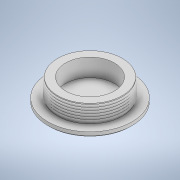
# Autodesk Inventor part: Abdeckung_Sensorkopfh
Saved by Autodesk Inventor 2022 (Build 260153000, 153)
## iProperties
Created: 2023-07-31
Part Number: Abdeckung_Sensorkopfh
Material: Generisch
Document SubType Name: Modeling
Designer: aewalder
Density: 1 g/cm^3
Appearance: Vorgabe
Author: aewalder
Autodesk Inventor part; units mm, degrees
ref_plane "YZ Plane" through (0, 0, 0) normal (1, 0, 0) x (0, 1, 0)
ref_plane "XZ Plane" through (0, 0, 0) normal (0, 1, 0) x (-1, 0, 0)
ref_plane "XY Plane" through (0, 0, 0) normal (0, 0, 1) x (1, 0, 0)
sketch "Sketch1" plane through (0, 0, 0) normal (0, 0, 1) x (1, 0, 0)
  line L0 (16, 0) -> (16, 1.8)
  line L1 (16, 1.8) -> (12.3, 1.8)
  line L2 (12.3, 1.8) -> (12.3, 2.4)
  arc A0 (12.3, 2.4) -> (12.3, 3.2) centre (12.3, 2.8) ccw
  line L3 (12.3, 3.2) -> (12.3, 3.4)
  arc A1 (12.3, 3.4) -> (12.3, 4.2) centre (12.3, 3.8) ccw
  line L4 (12.3, 4.2) -> (12.3, 4.4)
  arc A2 (12.3, 4.4) -> (12.3, 5.2) centre (12.3, 4.8) ccw
  line L5 (12.3, 5.2) -> (12.3, 8.6)
  line L6 (12.3, 8.6) -> (9.3, 8.6)
  line L7 (9.3, 8.6) -> (9.3, 1.8)
  line L8 (9.3, 1.8) -> (0, 1.8)
  line L9 (0, 1.8) -> (0, 0)
  line L10 (0, 0) -> (16, 0)
  line L11 (12.5, 4.8) -> (12.5, 2.8) construction
  line L12 (12.3, 4.8) -> (12.5, 4.8) construction
  line L13 (12.3, 2.8) -> (12.5, 2.8) construction
  line L14 (12.7, 4.8) -> (12.7, 2.8) construction
  line L15 (12.3, 5.8) -> (12.5, 5.8) construction
  arc A3 (12.3, 5.4) -> (12.3, 6.2) centre (12.3, 5.8) ccw
  line L16 (12.3, 6.8) -> (12.5, 6.8) construction
  arc A4 (12.3, 6.4) -> (12.3, 7.2) centre (12.3, 6.8) ccw
  line L17 (12.3, 7.8) -> (12.5, 7.8) construction
  arc A5 (12.3, 7.4) -> (12.3, 8.2) centre (12.3, 7.8) ccw
  point P0 (12.7, 5.8)
  point P1 (12.7, 6.8)
  point P2 (12.7, 7.8)
  point P3 (12.3, 8.2)
  point P4 (12.3, 7.4)
  point P5 (12.3, 6.2)
  point P6 (12.3, 5.4)
  point P7 (12.3, 7.2)
  point P8 (12.3, 6.4)
  dimension "d0" = 25
  dimension "d1" = 0.2
  dimension "d2" = 1
  dimension "d3" = 1
  dimension "d5" = 1
  dimension "d6" = 0.2
  dimension "d8" = 1.8
  dimension "d10" = 32
  dimension "d17" = 1
  dimension "d22" = 0.8
  dimension "d23" = 3
  constraints: 36 end point, 14 point on circle, 11 point on line, 6 centre point, 5 perpendicular, 3 horizontal, 3 vertical, 2 equal radius, 21 other
  measures "d0" diameter of L11 L9
  measures "d1" distance between parallel lines of L14 L11
  measures "d2" distance of L13.start A1.centre
  measures "d3" distance of L12.start A1.centre
  measures "d5" distance from line of L1 L13.start
  measures "d6" distance between parallel lines of L11 L4
  measures "d8" distance between parallel lines of L10 L1
  measures "d10" diameter of L0 L9
  measures "d17" distance of L12.start L15.start
  measures "d22" distance of L5.end L17.start
  measures "d23" distance between parallel lines of L7 L5
revolve "Revolution1" add sketch "Sketch1" angle 360 about axis through (0, 1.8, 0) along (0, -1, 0)
chamfer "Chamfer1" distance 0.5 angle 45 1 edges at (-16, 0, 0)
equation "\"d3\" = d2"
body "Solid1"
